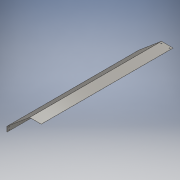
# Autodesk Inventor part: MC Part2b
Saved by Autodesk Inventor 2016 (Build 200138000, 138)
## iProperties
Created: 2017-11-07
Part Number: MC Part2b
Material: Steel, Mild
Document SubType Name: Sheet Metal
Designer: m207653
Density: 7.85 g/cm^3
Sheet Metal Rule: ms steel
Appearance: Semi-Polished
Flat Pattern Width: 59.3305 cm
Flat Pattern Length: 169.5 cm
Flat Pattern Area: 10056.5 cm^2
Sheet Metal Width: 593.305 mm
Sheet Metal Length: 1695.000 mm
Sheet Metal Area: 1005652.545 mm^2
Author: m207653
Autodesk Inventor part; units mm, degrees
ref_plane "YZ Plane" through (0, 0, 0) normal (1, 0, 0) x (0, 1, 0)
ref_plane "XZ Plane" through (0, 0, 0) normal (0, 1, 0) x (-1, 0, 0)
ref_plane "XY Plane" through (0, 0, 0) normal (0, 0, 1) x (1, 0, 0)
sketch "Sketch1" plane through (0, 0, 0) normal (0, 0, 1) x (1, 0, 0)
  line L0 (0, 0) -> (150, 0)
  line L1 (150, 0) -> (150, 1695)
  line L2 (150, 1695) -> (0, 1695)
  line L3 (0, 1695) -> (0, 0)
  dimension "d0" = 150
  dimension "d1" = 1695
  measures "d0" distance of L0.start L0.end
  measures "d1" distance of L0.end L1.end
extrude "Plate1" add sketch "Sketch1" along normal blind 1.6
sketch "Sketch2" plane through (1.0285, 0, 0.3743) normal (-0.6427876, 0, 0.7660444) x (0, -1, 0)
  line L0 (-1695, 0) -> (0, 0)
  line L1 (0, 0) -> (0, 380)
  line L2 (0, 380) -> (-1695, 380)
  line L3 (-1695, 380) -> (-1695, 0)
  constraints: 6 end point, 1 horizontal, 1 perpendicular, 1 vertical
edge flange "Flange1" height 380 angle 40 thickness 1.6 bend radius 1.6 thickness toward (-0.6427876, 0, 0.7660444) relief straight relief width 1.6 relief depth 0.8 edges at (0, 847.5, 1.6) wall of the first edge with corners at (1.0285, 1695, 0.3743) (1.0285, 0, 0.3743) (-290.0684, 0, -243.885) (-290.0684, 1695, -243.885)
bend "Bend1"
corner "Corner1"
sketch "Sketch3" plane through (-289.4969, 0, -242.6593) normal (-1, 0, 0) x (0, -1, 0)
  line L0 (-1695, 0) -> (0, 0)
  line L1 (0, 0) -> (0, 65)
  line L2 (0, 65) -> (-1695, 65)
  line L3 (-1695, 65) -> (-1695, 0)
  constraints: 6 end point, 1 horizontal, 1 perpendicular, 1 vertical
edge flange "Flange2" height 65 angle 50 thickness 1.6 bend radius 1.6 thickness toward (-1, 0, 0) relief straight relief width 1.6 relief depth 0.8 edges at (-291.0969, 847.5, -242.6593) wall of the first edge with corners at (-289.4969, 1695, -242.6593) (-289.4969, 0, -242.6593) (-289.4969, 0, -307.6593) (-289.4969, 1695, -307.6593)
bend "Bend2"
corner "Corner2"
sketch "Sketch4" plane through (-291.0969, 0, -307.6593) normal (-1, 0, 0) x (0, 0, 1)
  line L0 (63.5078, 0) -> (0, 0) projected
  line L1 (0, 0) -> (61.6833, 0)
  line L2 (61.6833, 0) -> (61.6833, 1695)
  line L3 (63.5078, 1695) -> (0, 1695) projected
  circle A0 centre (46.6833, 25) radius 6
  circle A1 centre (15, 25) radius 6
  line L4 (0, 1695) -> (0, 0) projected
  circle A2 centre (46.6833, 1670) radius 6
  circle A3 centre (15, 1670) radius 6
  point P0 (307.6593, 0)
  dimension "d24" = 12
  dimension "d26" = 25
  dimension "d27" = 15
  dimension "d28" = 12
  dimension "d29" = 15
  dimension "d30" = 12
  dimension "d31" = 12
  dimension "d32" = 25
  dimension "d33" = 25
  constraints: 4 centre point, 4 end point, 2 point on line, 1 perpendicular
  measures "d24" diameter of A0
  measures "d26" distance from line of L0 A0.centre
  measures "d27" distance from line of L2 A0.centre
  measures "d28" diameter of A1
  measures "d29" distance from line of L4 A1.centre
  measures "d30" diameter of A2
  measures "d31" diameter of A3
  measures "d32" distance from line of L3 A2.centre
  measures "d33" distance from line of L3 A3.centre
hole "Hole1" at (-291.0969, 25, -260.976) at (-291.0969, 25, -292.6593) at (-291.0969, 1670, -260.976) at (-291.0969, 1670, -292.6593) direction (1, 0, 0) diameter 12 end through all
sketch "Sketch5" plane through (0, 0, 1.6) normal (0, 0, 1) x (1, 0, 0)
  line L0 (1.1647, 1695) -> (150, 1695) projected
  line L1 (150, 1695) -> (5, 1695)
  line L2 (5, 1695) -> (5, 1375.4099)
  line L3 (1.1647, 1695) -> (1.1647, 0) projected
  circle A0 centre (130, 1670) radius 6
  line L4 (150, 0) -> (150, 1695) projected
  circle A1 centre (25, 1670) radius 6
  point P0 (0, 0)
  dimension "d42" = 12
  dimension "d43" = 25
  dimension "d44" = 20
  dimension "d45" = 12
  dimension "d46" = 20
  constraints: 4 end point, 2 centre point, 1 parallel, 1 point on line
  measures "d42" diameter of A0
  measures "d43" distance from line of L0 A0.centre
  measures "d44" distance from line of L4 A0.centre
  measures "d45" diameter of A1
  measures "d46" distance from line of L2 A1.centre
hole "Hole2" at (130, 1670, 1.6) at (25, 1670, 1.6) direction (0, 0, -1) diameter 12 end through all
equation "\"d39\" = Thickness"
equation "\"d52\" = Thickness"
equation "\"d3\" = BendReliefWidth"
equation "\"d4\" = BendReliefDepth"
equation "\"d5\" = MinimumRemnant"
equation "\"d6\" = BendRadius"
equation "\"d9\" = BendRadius"
equation "\"d10\" = CornerReliefSize"
equation "\"d11\" = GapSize"
equation "\"d12\" = JacobiRadiusSize"
equation "\"d13\" = BendReliefWidth"
equation "\"d14\" = BendReliefDepth"
equation "\"d15\" = MinimumRemnant"
equation "\"d16\" = BendRadius"
equation "\"d19\" = BendRadius"
equation "\"d20\" = CornerReliefSize"
equation "\"d21\" = GapSize"
equation "\"d22\" = JacobiRadiusSize"
equation "\"BendRadius\" = Thickness"
equation "\"BendReliefWidth\" = Thickness"
equation "\"BendReliefDepth\" = 0.5 * Thickness"
equation "\"CornerReliefSize\" = 4 * Thickness"
equation "\"MinimumRemnant\" = 2 * Thickness"
equation "\"TransitionRadius\" = BendRadius"
equation "\"JacobiRadiusSize\" = BendRadius"
equation "\"GapSize\" = Thickness"
equation "\"d2\" = BendRadius"
equation "\"Thickness\" = 1.6"
body "Solid1"
